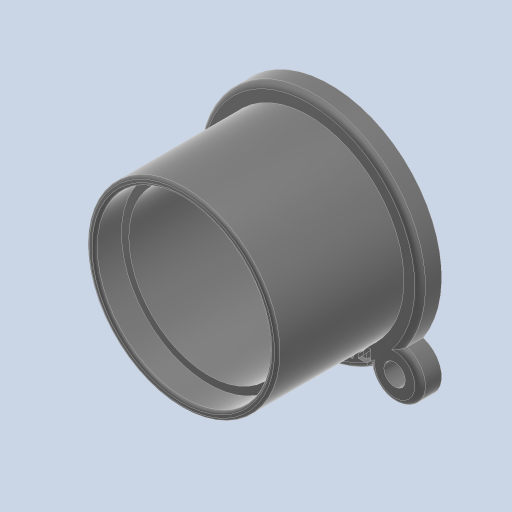
# Autodesk Inventor part: cage_outside_04
Saved by Autodesk Inventor 2024.4 (Build 284460000, 460)
## iProperties
Created: 2026-03-31
Part Number: cage_outside_04
Material: PLA Plastic
Document SubType Name: Modeling
Designer: tooles01
Density: 1.06 g/cm^3
Appearance: Smooth - White(2)
Author: tooles01
Autodesk Inventor part; units mm, degrees
ref_plane "YZ Plane" through (0, 0, 0) normal (1, 0, 0) x (0, 1, 0)
ref_plane "XZ Plane" through (0, 0, 0) normal (0, 1, 0) x (-1, 0, 0)
ref_plane "XY Plane" through (0, 0, 0) normal (0, 0, 1) x (1, 0, 0)
sketch "Sketch1: base" plane through (0, 0, 0) normal (0, 0, 1) x (1, 0, 0)
  circle A0 centre (33, 30) radius 16.25
  line L0 (17, 46) -> (17, 14) construction
  line L1 (17, 14) -> (49, 14) construction
  circle A1 centre (33, 30) radius 17.75
  circle A2 centre (17, 14) radius 1.8 construction
  circle A3 centre (17, 14) radius 3.25 construction
  circle A4 centre (49, 14) radius 1.8 construction
  circle A5 centre (49, 14) radius 3.25 construction
  circle A6 centre (33, 30) radius 20.75
  circle A7 centre (17, 14) radius 4.75
  circle A8 centre (49, 14) radius 4.75
  point P0 (0, 0)
  point P1 (50.3145, 18.5645)
  point P2 (15.6855, 18.5645)
  point P3 (21.5645, 12.6855)
  point P4 (44.4355, 12.6855)
  point P5 (17, 30)
  point P6 (33, 14)
  dimension "d4" = 32.5
  dimension "d18" = 1.5
  dimension "d32" = 3
  dimension "d33" = 1.5
  dimension "d34" = 6.5
  dimension "d35" = 3.6
  dimension "d36" = 32
  dimension "d37" = 32
  constraints: 9 centre point, 8 coincident, 4 end point, 3 equal radius, 2 midpoint, 1 horizontal, 1 horizontal alignment, 1 perpendicular, 1 vertical alignment, 1 other
  measures "d4" diameter of A0
  measures "d18" radial gap between concentric circles of A1 A0
  measures "d32" radial gap between concentric circles of A6 A1
  measures "d33" radial gap between concentric circles of A3 A7
  measures "d34" diameter of A3
  measures "d35" diameter of A2
  measures "d36" distance of L0.start L0.end
  measures "d37" distance of L0.end L1.end
extrude "Ex1: base" add sketch "Sketch1: base" along normal blind 4 contours A6 A8 A7 | A7 A6 | A6 A7 | A8 A6 | A6 A8
sketch "Sketch2: tube stopper" plane through (0, 0, 0) normal (0, 0, 1) x (1, 0, 0)
  circle A0 centre (33, 30) radius 14.875
  circle A1 centre (33, 30) radius 16.25 projected
  point P0 (0, 0)
  dimension "d22" = 29.75
  constraints: 1 centre point, 1 coincident
  measures "d22" diameter of A0
hole "Hole1: M3 inserts" at (49, 14, 0) at (17, 14, 0) direction (0, 0, 1) diameter 4 end through all
extrude "Ex2: tube cover" add sketch "Sketch1: base" along normal blind 27.6 contours A1
extrude "Ex3: tube stopper" add sketch "Sketch2: tube stopper" along normal blind 22.6
fillet "Fillet1: outside edges" radius 1 4 edges at (33, 50.75, 4) (52.3588, 10.6412, 4) (33, 9.25, 4) (13.6412, 10.6412, 4)
fillet "Fillet2: tube cover" radius 0.5 2 edges at (16.75, 30, 27.6) (15.25, 30, 27.6)
fillet "Fillet3: heat-set" [suppressed]
sketch "Sketch4: text" plane through (0, 0, 0) normal (0, 0, 1) x (1, 0, 0)
  line L0 (40.5, 16) -> (44, 16) construction
  line L1 (44, 16) -> (44, 12.5) construction
  line L2 (44, 12.5) -> (40.5, 12.5) construction
  line L3 (40.5, 12.5) -> (40.5, 16) construction
  line L4 (39.4248, 14.935) -> (40.3401, 14.935)
  line L5 (40.3401, 14.935) -> (40.7886, 13.4796)
  line L6 (40.7886, 13.4796) -> (41.2493, 14.935)
  line L7 (41.2493, 14.935) -> (42.1371, 14.935)
  line L8 (42.1371, 14.935) -> (41.1608, 12.6375)
  line L9 (41.1608, 12.6375) -> (40.3797, 12.6375)
  line L10 (40.3797, 12.6375) -> (39.4248, 14.935)
  line L11 (43.8213, 13.2294) -> (42.2164, 13.2294)
  line L12 (42.2164, 13.2294) -> (42.2164, 13.9556)
  line L13 (42.2164, 13.9556) -> (43.8213, 15.8625)
  line L14 (43.8213, 15.8625) -> (44.5901, 15.8625)
  line L15 (44.5901, 15.8625) -> (44.5901, 13.9129)
  line L16 (44.5901, 13.9129) -> (44.9868, 13.9129)
  line L17 (44.9868, 13.9129) -> (44.9868, 13.2294)
  line L18 (44.9868, 13.2294) -> (44.5901, 13.2294)
  line L19 (44.5901, 13.2294) -> (44.5901, 12.6375)
  line L20 (44.5901, 12.6375) -> (43.8213, 12.6375)
  line L21 (43.8213, 12.6375) -> (43.8213, 13.2294)
  line L22 (43.8213, 13.9129) -> (43.8213, 14.9136)
  line L23 (43.8213, 14.9136) -> (42.9731, 13.9129)
  line L24 (42.9731, 13.9129) -> (43.8213, 13.9129)
  point P0 (0, 0)
  point P1 (33, 30)
  dimension "d26" = 3.5
  dimension "d38" = 7.5
  dimension "d39" = 14
  constraints: 1 horizontal, 1 perpendicular, 2 other
  measures "d26" distance of L0.start L0.end
  measures "d38" distance from line of point (33, 30) L3
  measures "d39" distance from line of L0 point (33, 30)
extrude "Ex4: text" cut sketch "Sketch4: text" against normal blind 1 from surface at 4
body "Solid1"
